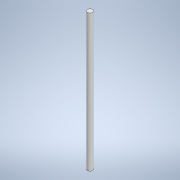
# Autodesk Inventor part: Rod_1
Saved by Autodesk Inventor 2022.3 (Build 263350000, 350)
## iProperties
Created: 2023-03-29
Part Number: Rod_1
Material: Generic
Document SubType Name: Modeling
Designer: Manuel Hueso Béjar
Density: 1 g/cm^3
Appearance: Default
Author: Manuel Hueso Béjar
Autodesk Inventor part; units mm, degrees
ref_plane "YZ Plane" through (0, 0, 0) normal (1, 0, 0) x (0, 1, 0)
ref_plane "XZ Plane" through (0, 0, 0) normal (0, 1, 0) x (-1, 0, 0)
ref_plane "XY Plane" through (0, 0, 0) normal (0, 0, 1) x (1, 0, 0)
sketch "Sketch1" plane through (0, 0, 0) normal (0, 1, 0) x (-1, 0, 0)
  circle A0 centre (0, 0) radius 4
  dimension "d0" = 8
  constraints: 1 centre point, 1 coincident
  measures "d0" diameter of A0
extrude "Extrusion1" add sketch "Sketch1" along normal blind 210
body "Solid1"
